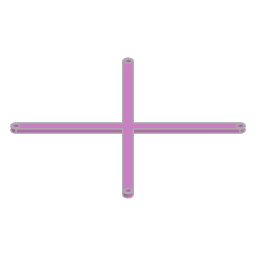
drone_ideal_model_symetry v2 (Autodesk Fusion 360 design; units mm, degrees)
Autodesk Fusion 360 part; units mm, degrees
note: some values were not read from the file. Set by a fixed rule: which sketch regions a step uses.
sketch "Szkic1" plane through (0, 0, 0) normal (0, 0, 1) x (1, 0, 0)
  circle A0 centre (0, 0) radius 63.5
  line L0 (0, 4.2415) -> (0, 63.5)
  line L1 (4.2415, 0) -> (63.5, 0)
  line L2 (42.78, 42.78) -> (44.9013, 44.9013)
  line L3 (42.78, -42.78) -> (44.9013, -44.9013)
  line L4 (-42.78, -42.78) -> (-44.9013, -44.9013)
  circle A1 centre (44.9013, 44.9013) radius 3
  line L5 (46.9719, 42.7304) -> (4.2415, 0)
  line L6 (42.7304, 46.9719) -> (0, 4.2415)
  line L7 (-42.7304, 46.9719) -> (0, 4.2415)
  line L8 (-46.9719, 42.7304) -> (-4.2415, 0)
  circle A2 centre (-44.9013, 44.9013) radius 3
  line L9 (46.9719, -42.7304) -> (4.2415, 0)
  line L10 (42.7304, -46.9719) -> (0, -4.2415)
  circle A3 centre (44.9013, -44.9013) radius 3
  line L11 (-42.7304, -46.9719) -> (0, -4.2415)
  line L12 (-46.9719, -42.7304) -> (-4.2415, 0)
  circle A4 centre (-44.9013, -44.9013) radius 3
  circle A5 centre (-44.9013, 44.9013) radius 2
  circle A6 centre (44.9013, 44.9013) radius 2
  circle A7 centre (44.9013, -44.9013) radius 2
  circle A8 centre (-44.9013, -44.9013) radius 2
  dimension "d2" = 135
  dimension "d3" = 6
  dimension "d4" = 4
  dimension "d5" = 4
  dimension "d6" = 4
  dimension "d7" = 4
  constraint coincident A0.centre origin
  constraint coincident A0 L0.end
  constraint vertical L0
  constraint coincident A0 L1.end
  constraint perpendicular L0 L1
  constraint symmetric L1 L2.end L3.end
  constraint coincident L2.end A1.centre
  constraint coincident A1 L5.start
  constraint coincident A0 L5.start
  constraint coincident A1 L6.start
  constraint coincident A0 L6.start
  constraint parallel L2 L6
  constraint parallel L2 L5
  constraint symmetric L0 A1 A2
  constraint symmetric L0 L5.start L8.start
  constraint symmetric L0 L6.start L7.start
  constraint symmetric L1 A1 A3
  constraint symmetric L1 L5.start L9.start
  constraint symmetric L1 L6.start L10.start
  constraint symmetric L1 L7.start L11.start
  constraint symmetric L1 L8.start L12.start
  constraint symmetric L1 A2 A4
  constraint concentric A2 A5
  constraint concentric A1 A6
  constraint coincident L3.end A3.centre
  constraint concentric A4 A8
  constraint coincident A3 L3.start
  constraint coincident A4 L4.start
  constraint coincident A1 L2.start
  measures "d2" angle of L1 L2
  measures "d3" diameter of A1
  measures "d4" diameter of A5
  measures "d5" diameter of A6
  measures "d6" diameter of A7
  measures "d7" diameter of A8
extrude "Wyciągnięcie proste1" add sketch "Szkic1" along normal blind 3 contours A0 L2 A1 A6 | A1 L5 L6 L7 L8 A2 L9 L10 A3 L11 L12 A4 | A0 A1 A6 | A0 A3 A7 | A0 L3 A3 A7 | A0 L2 A1 A6 | A0 L3 A3 A7 | A0 A4 A8 | A0 L4 A4 A8 | A0 A2 A5 | A0 A2 A5 | A0 L4 A4 A8
equation "d2 = 90 deg + 45 deg"
